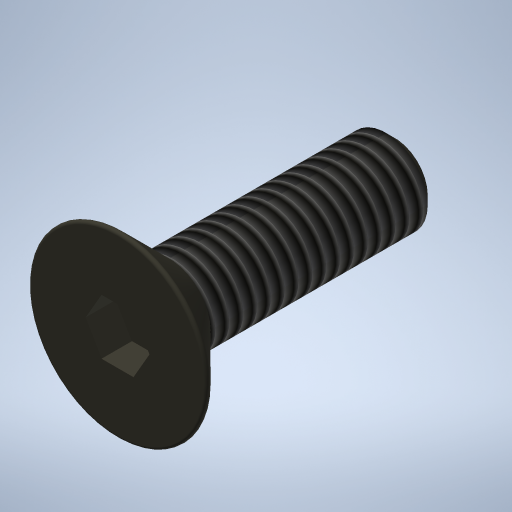
# Autodesk Inventor part: SCREW,FLAT-HD,P,10_9,M03X0_50X010MM
Saved by Autodesk Inventor 2024.3 (Build 283343000, 343)
## iProperties
ILogicPurgeVersion: 0.0.0.0
OnSaveVersion: 2.0.5.20
OnSaveAssembly: CLInventorObjectModel
Category: _
Manager: 100-30686
Created: 2024-07-12
Part Number: SCREW,FLAT-HD,P,10_9,M03X0_50X010MM
Checked By: 0004355540
Engr Approved By: P
User Status: Released
Material: Steel, MS
Description: SCREW,FLAT-HD,P,10.9,M03X0.50X010MM
Document SubType Name: Modeling
Mfg Approved By: Clint.Matte
Designer: Clint.Matte
Manufacturer: Standard
Standards Organization: Custom
Density: 7.86 g/cm^3
Appearance: Gunmetal
Mass: 0.70165 g
Surface Area: 1.60106 cm^2
Volume: 0.0892684 cm^3
CN_MASS: 0.0
CN_SERVICEABLE: _
FIRST_DESCRIPTION: FLAT HEAD SOCKET CAP SCREW, STEEL 10.9
SECOND_DESCRIPTION: M3 x 0.5 x 10 MM
THIRD_DESCRIPTION: WV
ModelCat: Uncategorized
PTC_WM_ITERATION: 3
PTC_WM_ORGANIZATION_ID: CLWC
PTC_WM_LIFECYCLE: CLWC_CAD_LC
Subject: FMPFH8A030050010
Author: Clint.Matte
Keywords: GENERIC
Revision Number: 1
Autodesk Inventor part; units mm, degrees
ref_plane "YZ Plane" through (0, 0, 0) normal (1, 0, 0) x (0, 1, 0)
ref_plane "XZ Plane" through (0, 0, 0) normal (0, 1, 0) x (-1, 0, 0)
ref_plane "XY Plane" through (0, 0, 0) normal (0, 0, 1) x (1, 0, 0)
sketch "Sketch2" plane through (0, 0, 0) normal (0, 0, 1) x (1, 0, 0)
  circle A0 centre (0, 0) radius 1.5
  dimension "Diameter" = 3
  constraints: 1 centre point, 1 coincident
  measures "Diameter" diameter of A0
extrude "Extrusion1" add sketch "Sketch2" against normal blind 8.14
sketch "Sketch3" plane through (0, 0, 0) normal (0, 0, 1) x (1, 0, 0)
  circle A0 centre (0, 0) radius 1.5 projected
extrude "Extrusion2" add sketch "Sketch3" along normal blind 1.86 draft 45
sketch "Sketch4" plane through (0, 0, 1.86) normal (0, 0, 1) x (1, 0, 0)
  circle A0 centre (0, 0) radius 3.36 projected
  line L0 (0.5774, 1) -> (1.1547, 0)
  line L1 (1.1547, 0) -> (0.5774, -1)
  line L2 (0.5774, -1) -> (-0.5774, -1)
  line L3 (-0.5774, -1) -> (-1.1547, 0)
  line L4 (-1.1547, 0) -> (-0.5774, 1)
  line L5 (-0.5774, 1) -> (0.5774, 1)
  line L6 (0, 0) -> (1.1547, 0) construction
  dimension "Hex_Width" = 2
  constraints: 14 end point, 1 coincident, 1 horizontal, 13 other
  measures "Hex_Width" distance between parallel lines of L0 L3
extrude "Extrusion3" cut sketch "Sketch4" against normal blind 1.1 contours L0 L1 L2 L3 L4 L5
thread "Thread1" size "M3x0.5" class "6g" standard "ANSI Metric M Profile-Short lst" length 8.14
chamfer "Chamfer1" distance 0.3 angle 45 1 edges at (-1.5, 0, -8.14)
fillet "Fillet1" radius 0.1 1 edges at (-3.36, 0, 1.86)
equation "\"Length1\" = Length - Head_Height"
equation "\"Thread_Length\" = Length1"
equation "\"Length\" = 10"
equation "\"Head_Height\" = 1.86"
body "Solid1"
